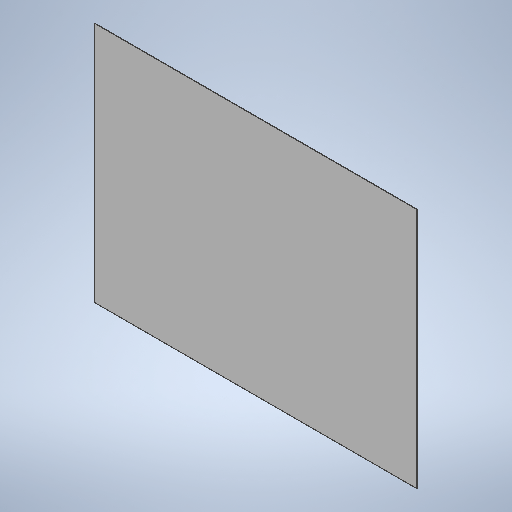
# Autodesk Inventor part: GBK-RK-0016 partition 6
Saved by Autodesk Inventor 2026.2 (Build 302298000, 298)
## iProperties
Created: 2026-09-14
Part Number: GBK-RK-0016 partition 6
Material: Generic
Document SubType Name: Sheet Metal
Designer: admin
Density: 1 g/cm^3
Sheet Metal Rule: Default_mm
Appearance: Default
Mass: 2973.5 g
Surface Area: 29844 cm^2
Volume: 2973.5 cm^3
Flat Pattern Width: 110 cm
Flat Pattern Length: 146.6 cm
Flat Pattern Area: 16126 cm^2
Sheet Metal Width: 1100,000 mm
Sheet Metal Length: 1466,000 mm
Sheet Metal Area: 1612600,000 mm^2
Author: admin
Autodesk Inventor part; units mm, degrees
ref_plane "YZ Plane" through (0, 0, 0) normal (1, 0, 0) x (0, 1, 0)
ref_plane "XZ Plane" through (0, 0, 0) normal (0, 1, 0) x (-1, 0, 0)
ref_plane "XY Plane" through (0, 0, 0) normal (0, 0, 1) x (1, 0, 0)
sketch "Sketch3" plane through (0, 0, 0) normal (0, 0, 1) x (1, 0, 0)
  line L0 (733, 1100) -> (733, 35.3553)
  line L1 (733, 35.3553) -> (697.6447, 0)
  line L2 (697.6447, 0) -> (-697.6447, 0)
  line L3 (-697.6447, 0) -> (-733, 35.3553)
  line L4 (-733, 35.3553) -> (-733, 1100)
  line L5 (-733, 1100) -> (733, 1100)
  line L6 (0, 0) -> (0, 1100) construction
  line L7 (673, 1100) -> (582.0074, 850)
  line L8 (582.0074, 850) -> (157.0074, 850)
  line L9 (157.0074, 850) -> (66.0149, 1100)
  line L10 (-66.0149, 1100) -> (-157.0074, 850)
  line L11 (-157.0074, 850) -> (-582.0074, 850)
  line L12 (-582.0074, 850) -> (-673, 1100)
  line L13 (-697.6447, 0) -> (-733, 0)
  line L14 (-733, 0) -> (-733, 35.3553)
  line L15 (697.6447, 0) -> (733, 0)
  line L16 (733, 0) -> (733, 35.3553)
  line L17 (-582.0074, 850) -> (-644.3394, 1100) construction
  line L18 (-369.5074, 1100) -> (-369.5074, 850) construction
  line L19 (-157.0074, 850) -> (-94.6754, 1100) construction
  dimension "d25" = 50
  dimension "d26" = 1100
  dimension "d27" = 1466
  dimension "d29" = 425
  dimension "d33" = 60
  dimension "d34" = 250
  dimension "d35" = 110
  dimension "d36" = 76
  dimension "d38" = 70
  dimension "d39" = 606.9851
  measures "d25" distance of L2.end L3.end
  measures "d27" distance of L4.end L0.start
  measures "d29" distance of L10.end L11.end
  measures "d33" distance of L12.end L4.end
  measures "d35" angle of L11 L12
  measures "d36" angle of L11 L19
  measures "d38" angle of L11 L10
  measures "d39" distance of L10.start L12.end
extrude "Plate3" add sketch "Sketch3" along normal blind 2
equation "\"d28\" = Thickness"
equation "\"BendRadius\" = Thickness"
equation "\"BendReliefWidth\" = Thickness"
equation "\"BendReliefDepth\" = 0.5 * Thickness"
equation "\"CornerReliefSize\" = 4 * Thickness"
equation "\"MinimumRemnant\" = 2 * Thickness"
equation "\"TransitionRadius\" = BendRadius"
equation "\"JacobiRadiusSize\" = BendRadius"
equation "\"GapSize\" = Thickness"
equation "\"Thickness\" = 2"
body "Solid2"
